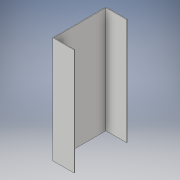
# Autodesk Inventor part: HopperRamp
Saved by Autodesk Inventor 2017 (Build 210142000, 142)
## iProperties
Created: 2020-02-22
Part Number: HopperRamp
Material: Generic
Document SubType Name: Modeling
Designer: S338674153
Density: 1 g/cm^3
Appearance: Default
Author: S338674153
Autodesk Inventor part; units mm, degrees
ref_plane "YZ Plane" through (0, 0, 0) normal (1, 0, 0) x (0, 1, 0)
ref_plane "XZ Plane" through (0, 0, 0) normal (0, 1, 0) x (-1, 0, 0)
ref_plane "XY Plane" through (0, 0, 0) normal (0, 0, 1) x (1, 0, 0)
sketch "Sketch1" plane through (0, 0, 0) normal (0, 1, 0) x (-1, 0, 0)
  line L0 (0, 0) -> (101.6, 0)
  line L1 (101.6, 0) -> (101.6, -4.2237)
  line L2 (98.425, -3.175) -> (0, -3.175)
  line L3 (0, -3.175) -> (0, 0)
  line L4 (101.6, 0) -> (6.8947, 0)
  line L5 (98.425, -3.175) -> (98.425, -250.825)
  line L6 (6.8947, -254) -> (101.6, -254)
  line L7 (101.6, -254) -> (101.6, 0)
  line L8 (101.6, -254) -> (0, -254)
  line L9 (0, -254) -> (0, -250.825)
  line L10 (0, -250.825) -> (98.425, -250.825)
  line L11 (101.6, -10.0234) -> (101.6, -254)
  dimension "d0" = 3.175
  dimension "d1" = 3.175
  dimension "d2" = 254
  dimension "d3" = 101.6
  constraints: 24 end point, 6 parallel, 3 horizontal, 3 perpendicular, 1 collinear, 1 point on line
  measures "d0" distance of L2.end L0.start
  measures "d1" distance between parallel lines of L5 L7
  measures "d2" distance of L6.end L0.end
  measures "d3" distance of L0.start L0.end
extrude "Extrusion1" add sketch "Sketch1" along normal blind 508
body "Solid1"
